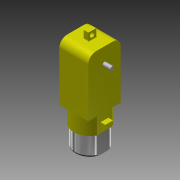
# Autodesk Inventor part: motor_dc
Saved by Autodesk Inventor 2015 (Build 190159000, 159)
## iProperties
Created: 2019-12-17
Part Number: motor_dc
Material: Generic
Document SubType Name: Modeling
Designer: Yuchofif
Density: 1 g/cm^3
Appearance: Default
Author: Yuchofif
Autodesk Inventor part; units mm, degrees
ref_plane "YZ Plane" through (0, 0, 0) normal (1, 0, 0) x (0, 1, 0)
ref_plane "XZ Plane" through (0, 0, 0) normal (0, 1, 0) x (-1, 0, 0)
ref_plane "XY Plane" through (0, 0, 0) normal (0, 0, 1) x (1, 0, 0)
sketch "Sketch1" plane through (0, 0, 0) normal (0, 1, 0) x (-1, 0, 0)
  line L0 (-9.33, 18.36) -> (9.33, 18.36)
  line L1 (9.33, 18.36) -> (9.33, -18.36)
  line L2 (9.33, -18.36) -> (-9.33, -18.36)
  line L3 (-9.33, -18.36) -> (-9.33, 18.36)
  line L4 (9.33, 18.36) -> (-9.33, -18.36) construction
  point P0 (0, 0)
  constraints: 10 end point, 2 parallel, 1 horizontal, 1 midpoint, 1 perpendicular
extrude "Extrusion1" add sketch "Sketch1" along normal blind 21
fillet "Fillet1" radius 5 2 edges at (0, 21, 18.36) (0, 0, 18.36)
sketch "Sketch2" plane through (9.33, 0, -18.36) normal (0, 0, -1) x (-1, 0, 0)
  circle A0 centre (9.33, 10.5) radius 10.5
  point P0 (9.33, 0)
  constraints: 1 centre point
extrude "Extrusion2" add sketch "Sketch2" along normal blind 10.7
sketch "Sketch3" plane through (9.33, 0, -18.36) normal (0, 0, 1) x (1, 0, 0)
  line L0 (0, 5.6832) -> (0, 15.3168) projected
  arc A0 (0, 5.6832) -> (0, 15.3168) centre (-9.33, 10.5) ccw projected
  line L1 (-18.66, 5.6832) -> (-18.66, 15.3168) projected
  arc A1 (-18.66, 15.3168) -> (-18.66, 5.6832) centre (-9.33, 10.5) ccw projected
  point P0 (-9.33, 0)
extrude "Extrusion3" cut sketch "Sketch3" against normal blind 10.7
sketch "Sketch4" plane through (9.33, 0, 13.36) normal (1, 0, 0) x (0, 0, -1)
  line L0 (36.17, 13) -> (38.67, 13)
  line L1 (38.67, 13) -> (38.67, 8)
  line L2 (38.67, 8) -> (36.17, 8)
  line L3 (36.17, 8) -> (36.17, 13)
  point P0 (13.36, 0)
  constraints: 8 end point, 2 parallel, 1 horizontal, 1 perpendicular
extrude "Extrusion4" add sketch "Sketch4" along normal blind 3
mirror "Mirror1" about plane through (0, 0, 0) normal (1, 0, 0) of "Extrusion4"
sketch "Sketch5" plane through (9.33, 0, -29.06) normal (0, 0, -1) x (-1, 0, 0)
  arc A0 (18.66, 15.3168) -> (0, 15.3168) centre (9.33, 10.5) ccw projected
  line L0 (0.83, 10.5) -> (0.83, 14.7426)
  line L1 (0.83, 10.5) -> (0.83, 6.2574)
  line L2 (9.33, 10.5) -> (9.33, 11.5651)
  line L3 (17.83, 10.5) -> (17.83, 14.7426)
  line L4 (17.83, 10.5) -> (17.83, 6.2574)
  arc A1 (17.83, 14.7426) -> (0.83, 14.7426) centre (9.33, 10.5) ccw
  arc A2 (0.83, 6.2574) -> (17.83, 6.2574) centre (9.33, 10.5) ccw
  point P0 (9.33, 0)
  point P1 (0.83, 15.6468)
  point P2 (0.83, 5.1568)
  point P3 (17.83, 15.6468)
  point P4 (17.83, 5.1568)
  constraints: 10 end point, 4 point on circle, 3 symmetric about line, 2 centre point, 1 coincident, 1 collinear, 1 parallel
extrude "Extrusion5" add sketch "Sketch5" along normal blind 12.74
fillet "Fillet2" radius 1 2 edges at (0, 20, -41.8) (0, 1, -41.8)
sketch "Sketch6" plane through (9.33, 0, -41.8) normal (0, 0, -1) x (-1, 0, 0)
  arc A0 (17.83, 10.5) -> (0.83, 10.5) centre (9.33, 10.5) ccw projected
  circle A1 centre (9.33, 10.5) radius 4.5
  point P0 (9.33, 0)
  dimension "d20" = 9
  constraints: 1 centre point, 1 coincident
  measures "d20" diameter of A1
extrude "Extrusion6" add sketch "Sketch6" along normal blind 2.5
fillet "Fillet3" radius 0.5 1 edges at (4.5, 10.5, -44.3)
sketch "Sketch7" plane through (0, 10.5, -44.3) normal (0, 0, -1) x (-1, 0, 0)
  circle A0 centre (0, 0) radius 4 projected
  circle A1 centre (0, 0) radius 4.5 projected
  circle A2 centre (0, 0) radius 4 projected
  line L0 (-3.0711, 4.7099) -> (3.07, 4.7099)
  line L1 (3.07, 4.7099) -> (3.07, 3.2901)
  line L2 (3.07, 3.2901) -> (-3.0711, 3.2901)
  line L3 (-3.0711, 3.2901) -> (-3.0711, 4.7099)
  line L4 (-3.0711, 4.7099) -> (3.07, 3.2901) construction
  line L5 (3.07, 4.7099) -> (-3.0711, 3.2901) construction
  point P0 (0, -10.5)
  point P1 (-0.0005, 4)
  constraints: 12 end point, 2 midpoint, 2 parallel, 1 horizontal, 1 perpendicular, 6 other
extrude "Extrusion7" cut sketch "Sketch7" against normal blind 2.5 contours L2 A0 | A0 L2 A1 | A1 L3 L0 L1 picked at (0.4734, 3.4399) picked at (1.9981, 3.6326)
sketch "Sketch8" plane through (9.33, 0, -44.3) normal (0, 0, -1) x (-1, 0, 0)
  arc A0 (7.0551, 13.7901) -> (11.6049, 13.7901) centre (9.33, 10.5) ccw projected
  circle A1 centre (9.33, 10.5) radius 0.5
  point P0 (9.33, 0)
  dimension "d26" = 1
  constraints: 1 centre point, 1 coincident
  measures "d26" diameter of A1
extrude "Extrusion8" add sketch "Sketch8" along normal blind 0.5
sketch "Sketch9" plane through (-9.33, 5, 18.36) normal (0, 0, 1) x (1, 0, 0)
  line L0 (7.83, 8) -> (10.83, 8)
  line L1 (10.83, 8) -> (10.83, 3)
  line L2 (10.83, 3) -> (7.83, 3)
  line L3 (7.83, 3) -> (7.83, 8)
  line L4 (7.83, 8) -> (10.83, 3) construction
  line L5 (10.83, 8) -> (7.83, 3) construction
  point P0 (9.33, -5)
  point P1 (9.33, 5.5)
  dimension "d29" = 3
  dimension "d30" = 5
  constraints: 12 end point, 2 midpoint, 2 parallel, 1 horizontal, 1 perpendicular
  measures "d29" distance of L1.end L2.end
  measures "d30" distance of L0.end L1.end
extrude "Extrusion9" add sketch "Sketch9" along normal blind 5
sketch "Sketch10" plane through (1.5, 8, 18.36) normal (1, 0, 0) x (0, 0, -1)
  circle A0 centre (-2.5, 2.5) radius 1.5
  point P0 (18.36, -8)
  dimension "d33" = 3
  constraints: 1 centre point
  measures "d33" diameter of A0
extrude "Extrusion10" cut sketch "Sketch10" against normal blind 5
fillet "Fillet4" radius 0.5 4 edges at (1.5, 10.5, 18.36) (0, 13, 18.36) (-1.5, 10.5, 18.36) (0, 8, 18.36)
sketch "Sketch11" plane through (9.33, 0, 13.36) normal (1, 0, 0) x (0, 0, -1)
  circle A0 centre (4.89, 10.5) radius 1.25
  point P0 (13.36, 0)
  constraints: 1 centre point
extrude "Extrusion11" add sketch "Sketch11" along normal blind 5
mirror "Mirror3" about plane through (0, 0, 0) normal (1, 0, 0) of "Extrusion11"
body "Solid1"
